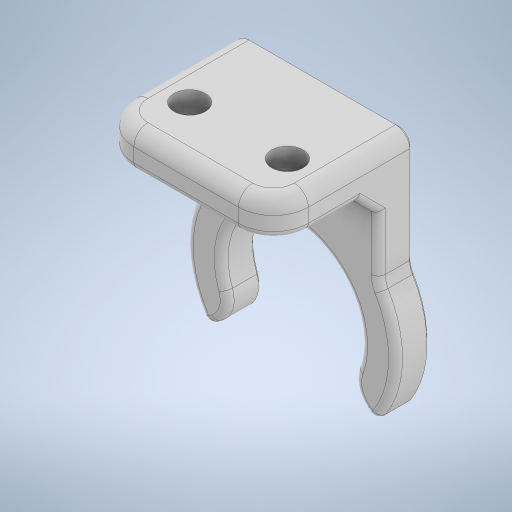
# Autodesk Inventor part: Teflon Holder Vertical V1
Saved by Autodesk Inventor 2023 (Build 270158000, 158)
## iProperties
Created: 2023-12-08
Part Number: Teflon Holder Vertical V1
Material: Generic
Document SubType Name: Modeling
Designer: Parker
Density: 1 g/cm^3
Appearance: Default
Author: Parker
Autodesk Inventor part; units mm, degrees
ref_plane "YZ Plane" through (0, 0, 0) normal (1, 0, 0) x (0, 1, 0)
ref_plane "XZ Plane" through (0, 0, 0) normal (0, 1, 0) x (-1, 0, 0)
ref_plane "XY Plane" through (0, 0, 0) normal (0, 0, 1) x (1, 0, 0)
sketch "Sketch1" plane through (0, 0, 0) normal (0, 0, 1) x (1, 0, 0)
  circle A0 centre (0, 0) radius 10
  circle A1 centre (0, 0) radius 15
  line L0 (0, 0) -> (-14.5417, -10.958)
  line L1 (0, 0) -> (14.3524, -10.8153)
  line L2 (0, 0) -> (0, -16.11)
  point P0 (7.9864, -6.0182)
  point P1 (11.9795, -9.0272)
  point P2 (-11.9795, -9.0272)
  point P3 (-7.9864, -6.0182)
  dimension "d0" = 20
  dimension "d1" = 30
  dimension "d2" = 53
  dimension "d3" = 53
  constraints: 6 end point, 2 centre point, 2 coincident, 1 vertical
  measures "d0" diameter of A0
  measures "d1" diameter of A1
  measures "d2" angle of L2 L0
  measures "d3" angle of L1 L2
extrude "Extrusion1" add sketch "Sketch1" along normal blind 5 contours A0 L0 A1 L1
sketch "Sketch2" plane through (0, 0, 5) normal (0, 0, 1) x (1, 0, 0)
  arc A0 (11.9795, -9.0272) -> (-11.9795, -9.0272) centre (0, 0) ccw projected
  line L0 (-11.9795, -9.0272) -> (-7.9864, -6.0182) projected
  arc A1 (7.9864, -6.0182) -> (-7.9864, -6.0182) centre (0, 0) ccw projected
  line L1 (7.9864, -6.0182) -> (11.9795, -9.0272) projected
  line L2 (-12.5, 20) -> (12.5, 20)
  line L3 (12.5, 20) -> (12.5, 10)
  line L4 (12.5, 10) -> (-12.5, 10)
  line L5 (-12.5, 10) -> (-12.5, 20)
  line L6 (-12.5, 20) -> (12.5, 10) construction
  line L7 (12.5, 20) -> (-12.5, 10) construction
  line L8 (-12.5, 10) -> (-12.5, 6.1508)
  line L9 (12.5, 10) -> (12.5, 4.604)
  point P0 (0, 15)
  point P1 (-12.5, 8.2916)
  point P2 (12.5, 8.2916)
  dimension "d6" = 25
  dimension "d7" = 10
  constraints: 16 end point, 2 midpoint, 2 parallel, 2 vertical, 1 horizontal, 1 perpendicular, 1 point on circle
  measures "d6" distance of L3.end L4.end
  measures "d7" distance of L2.end L3.end
extrude "Extrusion2" add sketch "Sketch2" against normal blind 5 contours A0 L4 L9 | A0 L4 L5 L2 L3 | A0 L8 L4
sketch "Sketch3" plane through (0, 0, 0) normal (0, 0, -1) x (-1, 0, 0)
  arc A0 (-12.5, 8.2916) -> (-11.9795, -9.0272) centre (0, 0) ccw projected
  line L0 (-7.9864, -6.0182) -> (-11.9795, -9.0272) projected
  arc A1 (7.9864, -6.0182) -> (-7.9864, -6.0182) centre (0, 0) ccw projected
  line L1 (11.9795, -9.0272) -> (7.9864, -6.0182) projected
  arc A2 (11.9795, -9.0272) -> (12.5, 8.2916) centre (0, 0) ccw projected
  line L2 (12.5, 8.2916) -> (12.5, 20) projected
  line L3 (12.5, 20) -> (-12.5, 20) projected
  line L4 (-12.5, 20) -> (-12.5, 8.2916) projected
  line L5 (-12.5, 20) -> (12.5, 20)
  line L6 (12.5, 20) -> (12.5, 25)
  line L7 (12.5, 25) -> (-12.5, 25)
  line L8 (-12.5, 25) -> (-12.5, 20)
  dimension "d10" = 25
  dimension "d11" = 5
  constraints: 8 end point, 2 parallel, 1 horizontal, 1 perpendicular
  measures "d10" distance of L7.end L6.end
  measures "d11" distance of L6.end L5.end
extrude "Extrusion3" add sketch "Sketch3" against normal blind 20 contours L8 L7 L6 L3
sketch "Sketch4" plane through (-12.5, 20, 5) normal (0, -1, 0) x (1, 0, 0)
  line L0 (0, 0) -> (0, 15) projected
  line L1 (0, 7.5) -> (25, 7.5)
  line L2 (25, -5) -> (25, 15) projected
  point P0 (12.5, -5)
  point P1 (12.5, 7.5)
  point P2 (5.5, 7.5)
  point P3 (19.5, 7.5)
  dimension "d14" = 7
  dimension "d15" = 7
  constraints: 3 point on line, 2 end point, 2 midpoint, 1 horizontal
  measures "d14" distance of point (12.5, 7.5) point (5.5, 7.5)
  measures "d15" distance of point (19.5, 7.5) point (12.5, 7.5)
hole "Hole1" at (-7, 20, 12.5) at (7, 20, 12.5) direction (0, 1, 0) diameter 4.5 end through all
chamfer "Chamfer1" distance 2 angle 45 2 edges at (-7, 20, 14.75) (7, 20, 14.75)
fillet "Fillet1" radius 5 2 edges at (-12.5, 22.5, 20) (12.5, 22.5, 20)
fillet "Fillet2" radius 4 2 edges at (-7.9864, -6.0182, 2.5) (7.9864, -6.0182, 2.5)
fillet "Fillet3" radius 1 2 edges at (-11.9795, -9.0272, 2.5) (11.9795, -9.0272, 2.5)
chamfer "Chamfer2" distance 3 angle 45 1 edges at (0, 20, 5)
fillet "Fillet4" radius 2 5 edges at (11.0355, 25, 18.5355) (0, 25, 20) (-11.0355, 25, 18.5355) (-12.5, 25, 7.5) (12.5, 25, 7.5)
fillet "Fillet5" radius 3 2 edges at (-12.5, 8.2916, 2.5) (12.5, 8.2916, 2.5)
chamfer "Chamfer3" distance 0.5 angle 45 16 edges at (-12.5, 16.0758, 0) (-11.9142, 24.4142, 0) (0, 25, 0) (11.9142, 24.4142, 0) (12.5, 16.0758, 0) (12.606, 8.3609, 0) (14.9969, -0.307, 0) (11.9286, -8.5899, 0) (10.9336, -8.239, 0) (9.2829, -6.0024, 0) (0, 10, 0) (-9.2829, -6.0024, 0) (-10.9336, -8.239, 0) (-11.9286, -8.5899, 0) (-14.9969, -0.307, 0) (-12.606, 8.3609, 0)
fillet "Fillet6" radius 1 20 edges at (-11.9286, -8.5899, 5) (-10.9336, -8.239, 5) (-9.2829, -6.0024, 5) (0, 10, 5) (9.2829, -6.0024, 5) (10.9336, -8.239, 5) (11.9286, -8.5899, 5) (14.9969, -0.307, 5) (12.606, 8.3609, 5) (12.5, 13.0758, 5) (-12.606, 8.3609, 5) (-12.5, 13.0758, 5) (-14.9969, -0.307, 5) (-12.5, 18.5, 6.5) (-11.0355, 20, 18.5355) (0, 20, 20) (11.0355, 20, 18.5355) (12.5, 20, 11.5) (-12.5, 20, 11.5) (12.5, 18.5, 6.5)
body "Solid1"
